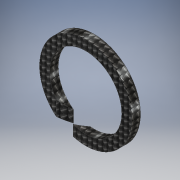
# Autodesk Inventor part: reverse gear piston gear
Saved by Autodesk Inventor 2017 (Build 210142000, 142)
## iProperties
Created: 2018-11-02
Part Number: reverse gear piston gear
Material: Generic
Document SubType Name: Modeling
Designer: User
Density: 1 g/cm^3
Appearance: Default
Author: User
Autodesk Inventor part; units mm, degrees
ref_plane "YZ Plane" through (0, 0, 0) normal (1, 0, 0) x (0, 1, 0)
ref_plane "XZ Plane" through (0, 0, 0) normal (0, 1, 0) x (-1, 0, 0)
ref_plane "XY Plane" through (0, 0, 0) normal (0, 0, 1) x (1, 0, 0)
sketch "Sketch1" plane through (0, 0, 0) normal (0, 1, 0) x (-1, 0, 0)
  circle A0 centre (0, 0) radius 16
  dimension "d74" = 32
  constraints: 1 centre point
  measures "d74" diameter of A0
extrude "Extrusion3" add sketch "Sketch1" along normal blind 3
sketch "Sketch4" plane through (0, 3, 0) normal (0, 1, 0) x (1, 0, 0)
  circle A0 centre (0, 0) radius 12.5
  line L0 (-4.3909, 10.9342) -> (-4.3909, 17.3914)
  line L1 (-4.3909, 17.3914) -> (-7.1862, 17.3914)
  line L2 (-7.1862, 17.3914) -> (-7.1862, 9.3059)
  line L3 (-7.1862, 9.3059) -> (-4.3909, 9.3059)
  line L4 (-4.3909, 9.3059) -> (-4.3909, 10.9342)
  dimension "d77" = 25
  constraints: 10 end point, 3 perpendicular, 1 centre point, 1 coincident, 1 horizontal, 1 vertical
  measures "d77" diameter of A0
extrude "Extrusion4" cut sketch "Sketch4" against normal through all
chamfer "Chamfer3" distance 3 angle 45 1 edges at (-4.3909, 3, -13.5446)
chamfer "Chamfer4" distance 3 angle 45 1 edges at (-7.1862, 0, -12.2616)
body "Solid3"
